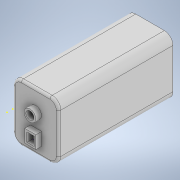
# Autodesk Inventor part: Battery
Saved by Autodesk Inventor 2020 (Build 240168000, 168)
## iProperties
Created: 2021-06-20
Part Number: Battery
Material: Generic
Document SubType Name: Modeling
Designer: pc
Density: 1 g/cm^3
Appearance: Default
Author: pc
Autodesk Inventor part; units mm, degrees
ref_plane "YZ Plane" through (0, 0, 0) normal (1, 0, 0) x (0, 1, 0)
ref_plane "XZ Plane" through (0, 0, 0) normal (0, 1, 0) x (-1, 0, 0)
ref_plane "XY Plane" through (0, 0, 0) normal (0, 0, 1) x (1, 0, 0)
sketch "Sketch1" plane through (0, 0, 0) normal (1, 0, 0) x (0, 1, 0)
  line L0 (6.527, 9.1506) -> (-6.173, 9.1506)
  line L1 (-6.173, 9.1506) -> (-6.173, -16.2494)
  line L2 (-6.173, -16.2494) -> (6.527, -16.2494)
  line L3 (6.527, -16.2494) -> (6.527, 9.1506)
  point P0 (0, 0)
  constraints: 8 end point, 2 parallel, 1 horizontal, 1 perpendicular
extrude "Extrusion1" add sketch "Sketch1" along normal blind 10.16
sketch "Sketch2" plane through (0, -6.173, 9.1506) normal (0, 0, 1) x (1, 0, 0)
  circle A0 centre (5.08, 8.1197) radius 0.9096
  circle A1 centre (5.08, 8.1197) radius 1.2864
  line L0 (4.2941, 4.7416) -> (6.0229, 4.7416)
  line L1 (6.0229, 4.7416) -> (6.0229, 2.6232)
  line L2 (6.0229, 2.6232) -> (4.2941, 2.6232)
  line L3 (4.2941, 2.6232) -> (4.2941, 4.7416)
  line L4 (3.9413, 5.0852) -> (6.4125, 5.0852)
  line L5 (6.4125, 5.0852) -> (6.4125, 2.2224)
  line L6 (6.4125, 2.2224) -> (3.9413, 2.2224)
  line L7 (3.9413, 2.2224) -> (3.9413, 5.0852)
  point P0 (0, 6.173)
  constraints: 16 end point, 4 parallel, 2 centre point, 2 horizontal, 2 perpendicular, 1 coincident
extrude "Extrusion2" add sketch "Sketch2" along normal blind 1.27 separate body contours A0 | A1 | L0 L1 L2 L3 | L4 L5 L6 L7
sketch "Sketch3" plane through (0, -6.173, 9.1506) normal (0, 0, 1) x (1, 0, 0)
  circle A0 centre (5.0656, 8.1486) radius 0.9611
  line L0 (4.2551, 4.6027) -> (6.0267, 4.6027)
  line L1 (6.0267, 4.6027) -> (6.0267, 2.6271)
  line L2 (6.0267, 2.6271) -> (4.2551, 2.6271)
  line L3 (4.2551, 2.6271) -> (4.2551, 4.6027)
  point P0 (0, 6.173)
  constraints: 8 end point, 2 parallel, 1 centre point, 1 horizontal, 1 perpendicular
sketch "Sketch4" plane through (0, -6.173, 9.1506) normal (0, 0, 1) x (1, 0, 0)
  point P0 (0, 6.173)
sketch "Sketch5" plane through (5.08, 1.9467, 10.4206) normal (0, 0, 1) x (1, 0, 0)
  circle A0 centre (0, 0) radius 0.8976
  point P0 (-5.08, -1.9467)
  constraints: 1 centre point
extrude "Extrusion3" cut sketch "Sketch5" against normal blind 1.27 bodies 2
sketch "Sketch6" plane through (0, -6.173, 10.4206) normal (0, 0, 1) x (1, 0, 0)
  point P0 (0, 6.173)
sketch "Sketch7" plane through (0, -6.173, 10.4206) normal (0, 0, 1) x (1, 0, 0)
  line L0 (4.4305, 4.6319) -> (6.0358, 4.6319)
  line L1 (6.0358, 4.6319) -> (6.0358, 2.6414)
  line L2 (6.0358, 2.6414) -> (4.4305, 2.6414)
  line L3 (4.4305, 2.6414) -> (4.4305, 4.6319)
  point P0 (0, 6.173)
  constraints: 8 end point, 2 parallel, 1 horizontal, 1 perpendicular
extrude "Extrusion4" cut sketch "Sketch7" against normal blind 1.27 bodies 2
fillet "Fillet1" radius 1.905 4 edges at (10.16, 6.527, -3.5494) (0, 6.527, -3.5494) (10.16, -6.173, -3.5494) (0, -6.173, -3.5494)
fillet "Fillet2" radius 0.508 8 edges at (9.602, -5.615, 9.1506) (5.08, -6.173, 9.1506) (0.558, -5.615, 9.1506) (0, 0.177, 9.1506) (0.558, 5.969, 9.1506) (5.08, 6.527, 9.1506) (9.602, 5.969, 9.1506) (10.16, 0.177, 9.1506)
body "Solid1"
body "Solid2"
